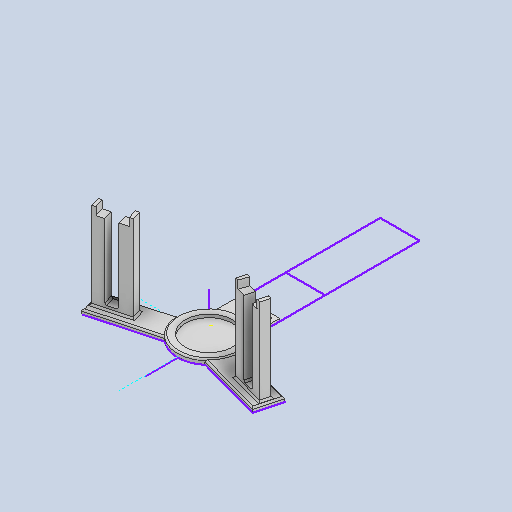
# Autodesk Inventor part: suporte_equipamento
Saved by Autodesk Inventor 2024.3 (Build 283343000, 343)
## iProperties
Created: 2024-12-04
Part Number: suporte_equipamento
Material: Genérico
Document SubType Name: Modeling
Designer: lostv
Density: 1 g/cm^3
Appearance: Padrão
Author: lostv
Autodesk Inventor part; units mm, degrees
ref_plane "YZ Plane" through (0, 0, 0) normal (1, 0, 0) x (0, 1, 0)
ref_plane "XZ Plane" through (0, 0, 0) normal (0, 1, 0) x (-1, 0, 0)
ref_plane "XY Plane" through (0, 0, 0) normal (0, 0, 1) x (1, 0, 0)
sketch "Esboço1" plane through (0, 0, 0) normal (0, 1, 0) x (-1, 0, 0)
  line L0 (-11.5672, 14.1285) -> (43.3072, -40.746)
  line L1 (-11.5672, 14.1285) -> (-11.5672, 126.1285) construction
  line L2 (-11.5672, 14.1285) -> (-11.5672, 129.1285) construction
  ellipse E0 centre (-11.5672, 14.1285) end of major axis (94.9328, 14.1285) minor radius 112 (91.2832, 43.1974) -> (91.2788, 43.2144) ccw
  line L3 (86.8207, 41.9965) -> (91.2788, 43.2144)
  line L4 (-11.5672, 14.1285) -> (66.037, 14.1285) construction
  line L5 (-11.5672, 94.6285) -> (-11.5672, 14.1285)
  line L6 (83.7115, 53.3777) -> (83.7095, 53.3848)
  line L7 (83.7095, 53.3848) -> (87.775, 54.4954)
  line L8 (-11.5672, 14.1285) -> (94.9328, 14.1285) construction
  line L9 (-11.5672, 14.1285) -> (97.9328, 14.1285) construction
  ellipse E1 centre (-11.5672, 14.1285) end of major axis (97.9328, 14.1285) minor radius 115 (94.1763, 43.9919) -> (90.6781, 55.2908) ccw
  line L10 (95.12, 56.5105) -> (98.2355, 45.1063)
  line L11 (53.5646, 45.0993) -> (56.68, 33.6953)
  line L12 (95.12, 56.5105) -> (53.5646, 45.0993)
  line L13 (56.68, 33.6953) -> (97.6298, 44.9402)
  ellipse E2 centre (-11.5672, 14.1285) end of major axis (63.4328, 14.1285) minor radius 80.5 (60.9042, 34.8552) -> (57.2585, 46.1136) ccw
  ellipse E3 centre (-11.5672, 14.1285) end of major axis (-121.0672, 14.1285) minor radius 115 (-113.8126, 55.2908) -> (-117.3107, 43.9919) ccw
  line L14 (-118.2544, 56.5105) -> (-121.3699, 45.1063)
  line L15 (-76.699, 45.0993) -> (-79.8144, 33.6953)
  line L16 (-118.2544, 56.5105) -> (-76.699, 45.0993)
  line L17 (-79.8144, 33.6953) -> (-120.7643, 44.9402)
  ellipse E4 centre (-11.5672, 14.1285) end of major axis (-86.5672, 14.1285) minor radius 80.5 (-80.3929, 46.1136) -> (-84.0386, 34.8552) ccw
  circle A0 centre (-11.5672, 14.1285) radius 30
  circle A1 centre (-11.5672, 14.1285) radius 40
  line L18 (96.6777, 50.8084) -> (24.6648, 31.0767) construction
  line L19 (96.6942, 67.4927) -> (105.5342, 35.3008)
  line L20 (105.5342, 35.3008) -> (28.4328, 14.1285)
  line L21 (96.6942, 67.4927) -> (14.0958, 44.8109)
  line L22 (-119.8287, 67.4927) -> (-128.6687, 35.3008)
  line L23 (-128.6687, 35.3008) -> (-51.5672, 14.1285)
  line L24 (-119.8287, 67.4927) -> (-37.2302, 44.8109)
  line L25 (98.2355, 45.1063) -> (97.6298, 44.9402)
  line L26 (-120.7643, 44.9402) -> (-121.3849, 45.1104)
  ellipse E5 centre (-11.5672, 14.1285) end of major axis (-121.0672, 14.1285) minor radius 115 (-113.8126, 55.2908) -> (-117.3107, 43.9919) ccw
  line L27 (-118.2544, 56.5105) -> (-121.3699, 45.1063)
  line L28 (-118.2544, 56.5105) -> (-76.699, 45.0993)
  line L29 (-79.8144, 33.6953) -> (-120.7643, 44.9402)
  line L30 (-121.3699, 45.1063) -> (-120.7643, 44.9402)
  line L31 (13.4328, -25.8715) -> (-36.5672, -25.8715)
  line L32 (-36.5672, -25.8715) -> (-36.5672, -107.8715)
  line L33 (-36.5672, -107.8715) -> (13.4328, -107.8715)
  line L34 (13.4328, -107.8715) -> (13.4328, -25.8715)
  line L35 (13.4328, -107.8715) -> (-36.5672, -107.8715)
  line L36 (-36.5672, -107.8715) -> (-36.5672, -227.8715)
  line L37 (-36.5672, -227.8715) -> (13.4328, -227.8715)
  line L38 (13.4328, -227.8715) -> (13.4328, -107.8715)
  line L39 (13.4328, -25.8715) -> (13.4328, -17.0965)
  line L40 (-36.5672, -25.8715) -> (-36.5672, -17.0965)
  line L41 (13.4328, -25.8715) -> (-36.5672, -25.8715)
  line L42 (-36.5672, -25.8715) -> (-36.5672, -50.8715)
  line L43 (-36.5672, -50.8715) -> (13.4328, -50.8715)
  line L44 (13.4328, -50.8715) -> (13.4328, -25.8715)
  circle A2 centre (7.4328, -44.8715) radius 1.5
  circle A3 centre (7.4328, -44.8715) radius 2.75
  circle A4 centre (-30.5672, -44.8715) radius 1.5
  circle A5 centre (-30.5672, -44.8715) radius 2.75
  line L45 (83.006, 40.9543) -> (83.0136, 40.9266)
  line L46 (67.8975, 49.0351) -> (71.028, 37.6353)
  line L47 (82.1192, 52.9404) -> (85.2496, 41.5406)
  line L48 (-91.032, 49.0351) -> (-94.1624, 37.6353)
  line L49 (-105.2536, 52.9404) -> (-108.3841, 41.5406)
  point P0 (0, 0)
  point P1 (-11.4623, 7.2636)
  point P2 (-108.6492, 41.6134)
  point P3 (-105.5188, 53.0133)
  point P4 (82.3843, 53.0133)
  point P5 (85.5148, 41.6134)
  point P6 (13.4328, -50.8715)
  dimension "d1" = 80.5
  dimension "d36" = 11.4042
  dimension "d37" = 11.404
  dimension "d38" = 60
  dimension "d39" = 80
  dimension "d55" = 0.076
  dimension "d56" = 0.076
  dimension "d58" = 122
  dimension "d59" = 120
  dimension "d61" = 50
  dimension "d62" = 25
  dimension "d65" = 25
  dimension "d66" = 50
  dimension "d69" = 3
  dimension "d70" = 6
  dimension "d71" = 6
  dimension "d72" = 5.5
  constraints: 100 end point, 20 point on line, 19 symmetric about line, 13 parallel, 7 coincident, 7 perpendicular, 6 centre point, 6 horizontal, 6 vertical, 5 point on circle, 1 midpoint, 1 tangent, 26 other
  measures "d1" distance of L5.start L5.end
  measures "d36" vertical distance of L10.start L10.end
  measures "d37" vertical distance of L11.start L11.end
  measures "d38" diameter of A0
  measures "d39" diameter of A1
  measures "d55" angle of L10 L19
  measures "d56" angle of L22 L14
  measures "d58" distance from line of L33 L5.end
  measures "d59" distance of L37.end L33.end
  measures "d61" distance between parallel lines of L36 L38
  measures "d62" distance between parallel lines of L34 L2
  measures "d65" distance between parallel lines of L43 L31
  measures "d66" distance of L42.end L43.end
  measures "d69" diameter of A2
  measures "d70" distance from line of L44 A2.centre
  measures "d71" distance from line of L43 A2.centre
  measures "d72" diameter of A3
extrude "Extrusão1" add sketch "Esboço1" along normal blind 6 contours A0 L5 A1 L0 | L0 A1 L5 A0
extrude "Extrusão2" add sketch "Esboço1" along normal blind 2 contours L5 A0 L0 | L0 A0 L5
extrude "Extrusão3" add sketch "Esboço1" along normal blind 5 contours A1 L21 L19 L20 | A1 L23 L22 L24 | L6 L7 L12 | L16 L49 L17 E3 | E3 L17 L26 L14 L16 | L16 L48 L17 L49 | L16 E4 L17 L48 | L16 L15 L17 E4
extrude "Extrusão6" add sketch "Esboço1" along normal blind 105 contours L12 E1 L13 L47 | L46 L13 E2 L12 | L16 L49 L17 E3 | L16 E4 L17 L48
extrude "Extrusão7" add sketch "Esboço1" along normal blind 115 contours L12 L10 L25 L13 E1 | E2 L13 L11 L12 | E3 L17 L26 L14 L16 | L16 L15 L17 E4
extrude "Extrusão10" add sketch "Esboço1" along normal blind 2.5 contours L39 L31 A1 | L31 L40 A1 | L31 L34 L43 L32
extrude "Extrusão11" add sketch "Esboço1" along normal blind 2.5 contours A3 | A5
extrude "Extrusão12" cut sketch "Esboço1" along normal blind 0.7 contours A3 | A5
extrude "Extrusão13" add sketch "Esboço1" along normal blind 10 contours L47 L13 L46 L12 | L16 L48 L17 L49
fillet "Arredondamento1" radius 2 7 edges at (90.1179, 5, 24.7147) (78.5295, 5, 56.1518) (124.2487, 5, 51.3968) (51.5672, 6, 14.1285) (-66.9835, 5, 24.7147) (-55.395, 5, 56.1518) (-101.1142, 5, 51.3968)
chamfer "Chanfro1" distance 2 angle 45 14 edges at (100.2893, 5, 39.3177) (121.0671, 5, 45.0233) (78.2567, 5, 39.3973) (106.8188, 10, 47.2405) (92.5972, 10, 43.3352) (119.8122, 5, 50.8084) (-55.1223, 5, 39.3973) (-77.1549, 5, 39.3177) (-97.9326, 5, 45.0233) (-83.6844, 10, 47.2405) (-69.4628, 10, 43.3352) (97.4767, 5, 50.8049) (-74.3423, 5, 50.8049) (-96.6777, 5, 50.8084)
